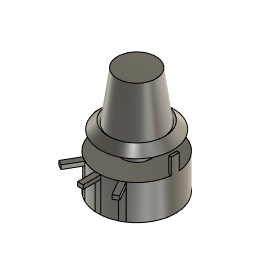
SPINDLE_BOX (Autodesk Fusion 360 archive; units mm, degrees)
design "spindle_control"
Autodesk Fusion 360 part; units mm, degrees
ref_plane "WorkPlane1" through (0, 0, 7) normal (0, 0, 1) x (1, 0, 0)
sketch "pot" plane through (0, 0, 0) normal (0, 0, 1) x (1, 0, 0)
  circle A0 centre (0, 0) radius 14.5
  circle A1 centre (0, 0) radius 5.25
  line L0 (13.5, 1.5) -> (15.5, 1.5)
  line L1 (15.5, 1.5) -> (15.5, -1.5)
  line L2 (15.5, -1.5) -> (13.5, -1.5)
  line L3 (13.5, -1.5) -> (13.5, 1.5)
  line L4 (13.5, 1.5) -> (15.5, -1.5) construction
  line L5 (15.5, 1.5) -> (13.5, -1.5) construction
  line L6 (-13.5, 1.5) -> (-15.5, 1.5)
  line L7 (-15.5, 1.5) -> (-15.5, -1.5)
  line L8 (-15.5, -1.5) -> (-13.5, -1.5)
  line L9 (-13.5, -1.5) -> (-13.5, 1.5)
  line L10 (-13.5, 1.5) -> (-15.5, -1.5) construction
  line L11 (-15.5, 1.5) -> (-13.5, -1.5) construction
  line L12 (-1.1104, -14.4574) -> (1, -14.4574)
  line L13 (1, -14.4574) -> (1, -21)
  line L14 (1, -21) -> (-1.1104, -21)
  line L15 (-1.1104, -21) -> (-1.1104, -14.4574)
  line L16 (-11.4617, -17.6313) -> (-8.1904, -11.9653)
  line L17 (-8.1904, -11.9653) -> (-6.3627, -13.0205)
  line L18 (-9.634, -18.6865) -> (-11.4617, -17.6313)
  line L19 (-6.3627, -13.0205) -> (-9.634, -18.6865)
  line L20 (9.5383, -18.7418) -> (6.267, -13.0757)
  line L21 (6.267, -13.0757) -> (8.0947, -12.0205)
  line L22 (8.0947, -12.0205) -> (11.366, -17.6865)
  line L23 (11.366, -17.6865) -> (9.5383, -18.7418)
  line L24 (0, 0) -> (-17.3232, 17.3232) construction
  line L25 (0, 0) -> (24.4987, 0) construction
  line L26 (-17.3232, 17.3232) -> (-18.596, 16.0504)
  line L27 (-17.3232, 17.3232) -> (-16.0504, 18.596)
  line L28 (-18.596, 16.0504) -> (-11.4465, 8.9009)
  line L29 (-16.0504, 18.596) -> (-8.9009, 11.4465)
  circle A2 centre (-16, 16) radius 1.25
  circle A3 centre (0, 0) radius 2.5
  point P0 (14.5, 0)
  point P1 (-14.5, 0)
  dimension "d1" = 29
  dimension "d2" = 10.5
  dimension "d3" = 2
  dimension "d4" = 3
  dimension "d5" = 2
  dimension "d6" = 3
  dimension "d7" = 135
  dimension "d8" = 1.8
  dimension "d9" = 1.8
  dimension "d10" = 2.5
  dimension "d14" = 5
  constraint coincident A0.centre A1.centre
  constraint horizontal L0
  constraint perpendicular L0 L1
  constraint parallel L0 L2
  constraint parallel L1 L3
  constraint coincident L4 P0
  constraint coincident L5 P0
  constraint coincident A0 P0
  constraint horizontal L6
  constraint perpendicular L6 L7
  constraint parallel L6 L8
  constraint parallel L7 L9
  constraint coincident L10 P1
  constraint coincident L11 P1
  constraint coincident A0 P1
  constraint horizontal L12
  constraint vertical L13
  constraint horizontal L14
  constraint vertical L15
  constraint coincident A0 L12.start
  constraint horizontal L25
  constraint perpendicular L24 L26
  constraint perpendicular L24 L27
  constraint coincident A0 L28.end
  constraint perpendicular L26 L28
  constraint coincident A0 L29.end
  constraint perpendicular L27 L29
  constraint coincident L24 A2.centre
  measures "d1" diameter of A0
  measures "d2" diameter of A1
  measures "d3" distance of L1.end L2.end
  measures "d4" distance of L0.end L1.end
  measures "d5" distance of L7.end L8.end
  measures "d6" distance of L6.end L7.end
  measures "d7" angle of L24 L25
  measures "d8" distance of L24.end L26.end
  measures "d9" distance of L24.end L27.end
  measures "d10" diameter of A2
  measures "d14" diameter of A3
sketch "knob" plane through (0, 0, 7) normal (0, 0, 1) x (1, 0, 0)
  circle A0 centre (0, 0) radius 13.5
  circle A1 centre (0, 0) radius 10
  circle A2 centre (0, 0) radius 7.5
  dimension "d11" = 27
  dimension "d12" = 20
  dimension "d13" = 15
  constraint coincident A0.centre A1.centre
  measures "d11" diameter of A0
  measures "d12" diameter of A1
  measures "d13" diameter of A2
extrude "Extrude1" add sketch "pot" against normal blind 13 contours A0 L0 L2 L3 L6 L8 L9 L12 L13 L17 L19 L21 L22 | A0 L0 L2 L3 | A0 L6 L8 L9 | A1 | A3 makes body 1
extrude "Extrude2" add sketch "pot" against normal blind 1.5 contours A0 L26 L27 L28 L29 | A0 L16 L18 L19 | A0 L20 L22 L23 | A0 L13 L14 L15 bodies 1
extrude "Extrude3" add sketch "pot" along normal blind 6 contours A0 L0 L2 L3 | A0 L6 L8 L9 bodies 1
extrude "Extrude4" add sketch "pot" along normal blind 20 contours A3 bodies 1
extrude "Extrude5" add sketch "pot" along normal blind 10 contours A1 bodies 1
extrude "Extrude6" add sketch "knob" along normal blind 20 draft -8 separate body contours A1 | A2 makes body 2
extrude "Extrude7" add sketch "knob" along normal blind 3 draft -45 contours A0 | A1 bodies 2

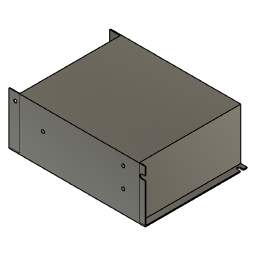
design "spindle_supply"
Autodesk Fusion 360 part; units mm, degrees
sketch "Sketch1" plane through (0, 0, 0) normal (0, 0, 1) x (1, 0, 0)
  line L0 (65, -48.5) -> (-65, -48.5)
  line L1 (-65, -48.5) -> (-65, 48.5)
  line L2 (-65, 48.5) -> (65, 48.5)
  line L3 (65, 48.5) -> (65, -48.5)
  line L4 (65, -48.5) -> (-65, 48.5) construction
  line L5 (-65, -48.5) -> (65, 48.5) construction
  line L6 (-65, 48.5) -> (2983, 48.5)
  line L7 (2983, 48.5) -> (2983, -49)
  line L8 (2983, -49) -> (-65, -49)
  line L9 (-65, -49) -> (-65, 48.5)
  line L10 (-65, 48.5) -> (-55, 48.5)
  line L11 (-55, 48.5) -> (-55, -49)
  line L12 (-55, -49) -> (-65, -49)
  line L13 (-65, -49) -> (-65, 48.5)
  line L14 (65, 48.5) -> (59, 48.5)
  line L15 (59, 48.5) -> (59, 38.5)
  line L16 (59, 38.5) -> (65, 38.5)
  line L17 (65, 38.5) -> (65, 48.5)
  line L18 (59, 38.5) -> (59, -49)
  line L19 (-65, 48.5) -> (59, 48.5)
  line L20 (59, 48.5) -> (59, 47.5)
  line L21 (59, 47.5) -> (-65, 47.5)
  line L22 (-65, 47.5) -> (-65, 48.5)
  line L23 (-65, -49) -> (65, -49)
  line L24 (65, -49) -> (65, -48)
  line L25 (65, -48) -> (-65, -48)
  line L26 (-65, -48) -> (-65, -49)
  line L27 (-56, 38) -> (-65, 38)
  line L28 (-65, 38) -> (-65, 23)
  line L29 (-65, 23) -> (-56, 23)
  line L30 (-56, 23) -> (-56, 38)
  line L31 (-56, -41) -> (-65, -41)
  line L32 (-65, -41) -> (-65, 14)
  line L33 (-65, 14) -> (-56, 14)
  line L34 (-56, 14) -> (-56, -41)
  line L35 (-65, 48.5) -> (-60, 48.5) construction
  line L36 (-60, 48.5) -> (-60, 43.5) construction
  circle A0 centre (-60, 43.5) radius 1.5
  line L37 (65, 48.5) -> (53, 48.5) construction
  line L38 (53, 48.5) -> (53, 41.5) construction
  circle A1 centre (53, 41.5) radius 1.5
  line L39 (65.5, 45) -> (62, 45)
  line L40 (65.5, 42) -> (62, 42)
  arc A2 (62, 45) -> (62, 42) centre (62, 43.5) ccw
  line L41 (-65, 48.5) -> (12.5, 48.5) construction
  line L42 (12.5, 48.5) -> (12.5, 18.5) construction
  line L43 (12.5, 18.5) -> (12.5, -14.5) construction
  circle A3 centre (12.5, 18.5) radius 1.5
  circle A4 centre (12.5, -14.5) radius 1.5
  line L44 (-65, -48.5) -> (-60, -48.5) construction
  line L45 (-60, -48.5) -> (-60, -43.5) construction
  circle A5 centre (-60, -43.5) radius 1.5
  dimension "d1" = 130
  dimension "d2" = 97
  dimension "d3" = 3048
  dimension "d4" = 10
  dimension "d5" = 6
  dimension "d6" = 10
  dimension "d7" = 1
  dimension "d8" = 1
  dimension "d9" = 15
  dimension "d10" = 55
  dimension "d11" = 5
  dimension "d12" = 5
  dimension "d13" = 3
  dimension "d14" = 12
  dimension "d15" = 7
  dimension "d16" = 3
  dimension "d17" = 77.5
  dimension "d18" = 30
  dimension "d19" = 33
  dimension "d20" = 3
  dimension "d21" = 3
  dimension "d22" = 5
  dimension "d23" = 5
  dimension "d24" = 3
  constraint horizontal L0
  constraint perpendicular L0 L1
  constraint parallel L0 L2
  constraint parallel L1 L3
  constraint coincident L4 origin
  constraint coincident L5 origin
  constraint horizontal L6
  constraint vertical L7
  constraint horizontal L8
  constraint vertical L9
  constraint horizontal L10
  constraint vertical L11
  constraint horizontal L12
  constraint vertical L13
  constraint horizontal L14
  constraint vertical L15
  constraint horizontal L16
  constraint vertical L17
  constraint perpendicular L0 L18
  constraint horizontal L19
  constraint vertical L20
  constraint horizontal L21
  constraint vertical L22
  constraint horizontal L23
  constraint vertical L24
  constraint horizontal L25
  constraint vertical L26
  constraint horizontal L27
  constraint vertical L28
  constraint horizontal L29
  constraint vertical L30
  constraint horizontal L31
  constraint vertical L32
  constraint horizontal L33
  constraint vertical L34
  constraint coincident L13 L32.end
  constraint perpendicular L1 L35
  constraint perpendicular L21 L36
  constraint coincident L36.end A0.centre
  constraint perpendicular L3 L37
  constraint perpendicular L21 L38
  constraint coincident L38.end A1.centre
  constraint perpendicular L17 L39
  constraint perpendicular L17 L40
  constraint tangent L40 A2
  constraint perpendicular L1 L41
  constraint perpendicular L21 L42
  constraint parallel L42 L43
  constraint coincident L42.end L43.start
  constraint coincident L43.end A4.centre
  constraint perpendicular L13 L44
  constraint perpendicular L31 L45
  constraint coincident L45.end A5.centre
  measures "d1" distance of L1.end L2.end
  measures "d2" distance of L0.end L1.end
  measures "d3" distance of L1.end L6.end
  measures "d4" distance of L1.end L10.end
  measures "d5" distance of L2.end L14.end
  measures "d6" distance of L2.end L16.end
  measures "d7" distance of L1.end L21.end
  measures "d8" distance of L8.end L25.end
  measures "d9" distance of L27.start L29.end
  measures "d10" distance of L31.start L33.end
  measures "d11" distance of L1.end L35.end
  measures "d12" distance of L35.end L36.end
  measures "d13" diameter of A0
  measures "d14" distance of L2.end L37.end
  measures "d15" distance of L37.end L38.end
  measures "d16" diameter of A1
  measures "d17" distance of L1.end L41.end
  measures "d18" distance of L41.end L42.end
  measures "d19" distance of L42.end L43.end
  measures "d20" diameter of A3
  measures "d21" diameter of A4
  measures "d22" distance of L0.end L44.end
  measures "d23" distance of L44.end L45.end
  measures "d24" diameter of A5
extrude "Extrude1" add sketch "Sketch1" along normal blind 50 contours L0 L3 L18 L24 L25 | L0 L11 L18 L25 | L0 L1 L9 L11 L13 L25 L26 | L11 L15 L18 L21 L25 | L1 L2 L6 L9 L10 L11 L13 L19 L21 L22 | L2 L6 L11 L15 L19 L20 L21 | A1 | A3 | A4 makes body 1
extrude "Extrude2" add sketch "Sketch1" along normal blind 20 separate body contours L1 L9 L13 L31 L32 L33 L34 | L1 L9 L13 L27 L28 L29 L30 makes body 2 at (-65, -22.6667, 6.6667) makes body 3 at (-56, 28, 6.6667)
extrude "Extrude3" add sketch "Sketch1" along normal blind 1 contours L3 L16 L18 L25 | L2 L3 L6 L14 L15 L16 L17 L20 L39 L40 A2 | L1 L9 L11 L13 L21 L25 L27 L29 L30 L31 L33 L34 bodies 1 2 3
extrude "Extrude4" cut sketch "Sketch1" along normal blind 5 contours A1 | A3 | A4 bodies 1
sketch "Sketch2" plane through (0, -48.5, 0) normal (0, -1, 0) x (1, 0, 0)
  line L0 (-65, 0) -> (65, 0)
  line L1 (65, 0) -> (65, 50)
  line L2 (65, 50) -> (-65, 50)
  line L3 (-65, 50) -> (-65, 0)
  line L4 (-65, 50) -> (65, 50)
  line L5 (-65, 0) -> (-65, 50)
  line L6 (65, 0) -> (-65, 0)
  line L7 (65, 0) -> (65, 50)
  line L8 (-65, 50) -> (-59, 50) construction
  line L9 (-59, 50) -> (-59, 42) construction
  circle A0 centre (-59, 42) radius 1.5
  line L10 (65, 50) -> (65, 40) construction
  line L11 (65, 38) -> (62, 38)
  line L12 (65, 42) -> (62, 42)
  arc A1 (62, 42) -> (62, 38) centre (62, 40) ccw
  line L13 (-65, 50) -> (-32.5, 50) construction
  line L14 (-32.5, 50) -> (-32.5, 30) construction
  line L15 (65, 50) -> (44, 50) construction
  line L16 (44, 50) -> (44, 40) construction
  line L17 (44, 40) -> (44, 21) construction
  circle A2 centre (-32.5, 30) radius 1.5
  circle A3 centre (44, 40) radius 1.5
  circle A4 centre (44, 21) radius 1.5
  dimension "d33" = 6
  dimension "d34" = 8
  dimension "d35" = 3
  dimension "d36" = 10
  dimension "d37" = 32.5
  dimension "d38" = 20
  dimension "d39" = 21
  dimension "d40" = 10
  dimension "d41" = 19
  dimension "d42" = 3
  dimension "d43" = 3
  dimension "d44" = 3
  constraint coincident L2.end L3.start
  constraint perpendicular L5 L8
  constraint perpendicular L8 L9
  constraint coincident L9.end A0.centre
  constraint coincident L1.end L2.start
  constraint coincident L1 L10.end
  constraint coincident L1 L11.start
  constraint perpendicular L7 L11
  constraint coincident L1 L12.start
  constraint perpendicular L10 L12
  constraint tangent L12 A1
  constraint tangent L11 A1
  constraint perpendicular L5 L13
  constraint perpendicular L4 L14
  constraint perpendicular L1 L15
  constraint perpendicular L2 L16
  constraint perpendicular L15 L17
  constraint coincident L14.end A2.centre
  constraint coincident L16.end L17.start
  constraint coincident L17.end A4.centre
  measures "d33" distance of L2.end L8.end
  measures "d34" distance of L8.end L9.end
  measures "d35" diameter of A0
  measures "d36" distance of L1.end L10.end
  measures "d37" distance of L2.end L13.end
  measures "d38" distance of L13.end L14.end
  measures "d39" distance of L1.end L15.end
  measures "d40" distance of L15.end L16.end
  measures "d41" distance of L16.end L17.end
  measures "d42" diameter of A2
  measures "d43" diameter of A3
  measures "d44" diameter of A4
extrude "Extrude5" cut sketch "Sketch2" against normal blind 5 contours L1 L7 L11 L12 A1 | A0 | A2 | A3 | A4 bodies 1
equation "d3 = 10'-0\""

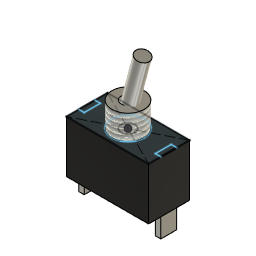
design "switch"
Autodesk Fusion 360 part; units mm, degrees
sketch "Sketch1" plane through (0, 0, 0) normal (0, 0, 1) x (1, 0, 0)
  line L0 (15, 7.5) -> (-15, 7.5)
  line L1 (-15, 7.5) -> (-15, -7.5)
  line L2 (-15, -7.5) -> (15, -7.5)
  line L3 (15, -7.5) -> (15, 7.5)
  line L4 (15, 7.5) -> (-15, -7.5) construction
  line L5 (-15, 7.5) -> (15, -7.5) construction
  circle A0 centre (0, 0) radius 6
  circle A1 centre (0, 0) radius 2.5
  line L6 (-15, 2.8547) -> (-13, 2.8547)
  line L7 (-13, 2.8547) -> (-13, -3)
  line L8 (-13, -3) -> (-15, -3)
  line L9 (-15, -3) -> (-15, 2.8547)
  line L10 (15, 2.7936) -> (13, 2.7936)
  line L11 (13, 2.7936) -> (13, -3)
  line L12 (13, -3) -> (15, -3)
  line L13 (15, -3) -> (15, 2.7936)
  dimension "d1" = 30
  dimension "d2" = 15
  dimension "d3" = 12
  dimension "d4" = 5
  constraint horizontal L0
  constraint perpendicular L0 L1
  constraint parallel L0 L2
  constraint parallel L1 L3
  constraint coincident L4 A0.centre
  constraint coincident L5 A0.centre
  constraint coincident A0.centre A1.centre
  constraint horizontal L6
  constraint vertical L7
  constraint horizontal L8
  constraint vertical L9
  constraint coincident L1 L6.start
  constraint horizontal L10
  constraint vertical L11
  constraint horizontal L12
  constraint vertical L13
  constraint coincident L3 L10.start
  measures "d1" distance of L1.end L2.end
  measures "d2" distance of L0.end L1.end
  measures "d3" diameter of A0
  measures "d4" diameter of A1
extrude "Extrude1" add sketch "Sketch1" along normal blind -26 and the other way blind 19 contours L3 L10 L11 L12 L13 | L1 L6 L7 L8 L9 makes body 1 at (-13, 0.9031, -21.3333) makes body 2 at (15, -1.0688, -21.3333)
extrude "Extrude2" add sketch "Sketch1" against normal blind 19 separate body contours L0 L1 L2 L3 L6 L7 L8 L10 L11 L12 | L3 L10 L11 L12 L13 | L1 L6 L7 L8 L9 | A0 | A1 makes body 3
extrude "Extrude3" add sketch "Sketch1" along normal blind 27 and the other way blind -6 separate body contours A1 makes body 4
extrude "Extrude4" add sketch "Sketch1" along normal blind 9 separate body contours A0 makes body 5
thread "Thread1" "ISO Metric profile 12.0 M12x1.75 6g" major diameter 11.8335 minor diameter 9.8365 pitch 1.75 angle 60 resizes the face on face at (5.9925, -0.2991, 6) on bodies 5
move_body "Move1" bodies 4 to x (0.965926, 0, -0.258819) y (0, 1, 0) z (0.258819, 0, 0.965926) at (-1.6381, 0, -0.4426)
